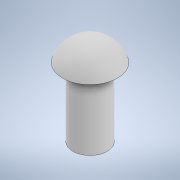
# Autodesk Inventor part: DERKS Hitch Peg
Saved by Autodesk Inventor 2020 (Build 240168000, 168)
## iProperties
Created: 2020-04-30
Part Number: DERKS Hitch Peg
Material: Generic
Document SubType Name: Modeling
Designer: tader
Density: 1 g/cm^3
Appearance: Default
Author: tader
Autodesk Inventor part; units mm, degrees
ref_plane "YZ Plane" through (0, 0, 0) normal (1, 0, 0) x (0, 1, 0)
ref_plane "XZ Plane" through (0, 0, 0) normal (0, 1, 0) x (-1, 0, 0)
ref_plane "XY Plane" through (0, 0, 0) normal (0, 0, 1) x (1, 0, 0)
sketch "Sketch1" plane through (0, 0, 0) normal (0, 0, 1) x (1, 0, 0)
  line L0 (0, 0) -> (0, 16.51)
  line L1 (0, 0) -> (3.175, 0)
  line L2 (3.175, 0) -> (3.175, 12.7)
  line L3 (3.175, 12.7) -> (5.08, 12.7)
  arc A0 (5.08, 12.7) -> (0, 16.51) centre (0.0064, 11.2268) ccw
  dimension "d0" = 16.51
  dimension "d1" = 3.175
  dimension "d2" = 12.7
  dimension "d3" = 1.905
  dimension "d4" = 5.2832
  constraints: 8 end point, 2 horizontal, 2 point on circle, 1 centre point, 1 perpendicular, 1 vertical
  measures "d0" distance of L0.start L0.end
  measures "d1" distance of L0.start L1.end
  measures "d2" distance of L1.end L2.end
  measures "d3" distance of L2.end L3.end
  measures "d4" radius of A0
revolve "Revolution1" add sketch "Sketch1" angle 360 about axis through (0, 0, 0) along (0, 1, 0)
body "Solid1"
